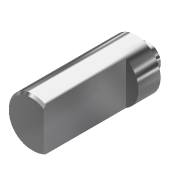
# Autodesk Inventor part: shaft_encoder
Saved by Autodesk Inventor 2014 (Build 180170000, 170)
## iProperties
Created: 2015-11-19
Part Number: shaft_encoder
Material: Generic
Document SubType Name: Modeling
Designer: Tom
Density: 1 g/cm^3
Appearance: Default
Author: Tom
Autodesk Inventor part; units mm, degrees
ref_plane "YZ Plane" through (0, 0, 0) normal (1, 0, 0) x (0, 1, 0)
ref_plane "XZ Plane" through (0, 0, 0) normal (0, 1, 0) x (-1, 0, 0)
ref_plane "XY Plane" through (0, 0, 0) normal (0, 0, 1) x (1, 0, 0)
sketch "Sketch1" plane through (0, 0, 0) normal (0, 0, 1) x (1, 0, 0)
  circle A0 centre (0, 0) radius 2.9845
  dimension "d0" = 5.969
  constraints: 1 centre point, 1 coincident
  measures "d0" diameter of A0
extrude "Extrusion1" add sketch "Sketch1" along normal blind 12.7
sketch "Sketch2" plane through (0, 0, 12.7) normal (0, 0, 1) x (1, 0, 0)
  circle A0 centre (0, 0) radius 2.9845 projected
  circle A1 centre (0, 0) radius 2.9845 projected
  line L0 (1.4859, 2.5883) -> (1.4859, -2.5883)
  dimension "d3" = 1.4859
  constraints: 2 end point, 2 point on circle, 1 vertical, 2 other
  measures "d3" distance from line of L0 point (0, 0)
extrude "Extrusion2" cut sketch "Sketch2" against normal blind 10.0076 contours A0 L0 picked at (1.9854, 0)
sketch "Sketch3" plane through (0, 0, 0) normal (0, 0, -1) x (-1, 0, 0)
  circle A0 centre (0, 0) radius 2.9845 projected
  circle A1 centre (0, 0) radius 1.4859
  constraints: 1 centre point, 1 coincident
extrude "Extrusion3" add sketch "Sketch3" along normal blind 1.524 contours A1
chamfer "Chamfer1" distance 0.254 angle 45 1 edges at (-2.9845, 0, 12.7)
body "Solid1"
